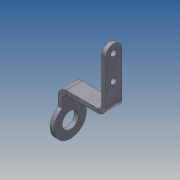
# Autodesk Inventor part: Gashebel_ra8846s
Saved by Autodesk Inventor 2021 (Build 250183000, 183)
## iProperties
Created: 2021-01-02
Part Number: Gashebel_ra8846s
Material: Aluminum 6061, geschweißt
Document SubType Name: Sheet Metal
Designer: Ricardo
Density: 2.7 g/cm^3
Sheet Metal Rule: Standard_mm
Appearance: Schweißnaht - Aluminum
Project: Motor
Description: Gashebel
Mass: 0.38312 g
Surface Area: 3.84459 cm^2
Volume: 0.141896 cm^3
Author: Sander
Revision Number: Rev00^
Autodesk Inventor part; units mm, degrees
ref_plane "YZ Plane" through (0, 0, 0) normal (1, 0, 0) x (0, 1, 0)
ref_plane "XZ Plane" through (0, 0, 0) normal (0, 1, 0) x (-1, 0, 0)
ref_plane "XY Plane" through (0, 0, 0) normal (0, 0, 1) x (1, 0, 0)
sketch "Skizze1" plane through (0, 0, 0) normal (0, 0, 1) x (1, 0, 0)
  line L0 (-38, 0) -> (11, 0)
  line L1 (0, -5.6) -> (0, 5.6)
  circle A0 centre (0, 0) radius 2
  line L2 (-3.4641, -2) -> (-29, -2)
  line L3 (-3.4641, 2) -> (-29, 2)
  arc A1 (-29, 2) -> (-29, -2) centre (-29, 0) ccw
  arc A2 (-3.4641, -2) -> (-3.4641, 2) centre (0, 0) ccw
  circle A3 centre (-29, 0) radius 0.75
  circle A4 centre (-23, 0) radius 0.75
  dimension "d0" = 4
  dimension "d1" = 4
  dimension "d2" = 6
  dimension "d3" = 1.5
  dimension "d4" = 1.5
  dimension "d5" = 2
  dimension "d6" = 29
  measures "d0" diameter of A0
  measures "d1" radius of A2
  measures "d2" distance of A1.centre A4.centre
  measures "d3" diameter of A4
  measures "d4" diameter of A3
  measures "d5" radius of A1
  measures "d6" distance from line of L1 A1.centre
extrude "Grobblech1" add sketch "Skizze1" along normal blind 1 contours A1 L3 A2 L1 A0 L0 A4 A3 | L0 A3 A4 A0 L1 A2 L2 A1 | A2 L0 A0 L1 | L1 A0 L0 A2
sketch "Skizze2" plane through (0, 0, 1) normal (0, 0, 1) x (1, 0, 0)
  circle A0 centre (-29, 0) radius 0.75 projected
  line L0 (-3.4641, -2) -> (-29, -2) projected
  line L1 (-29, 2) -> (-3.4641, 2) projected
  line L2 (-7, 2) -> (-7, -2)
  dimension "d8" = 22
  constraints: 2 end point, 2 point on line, 1 perpendicular
  measures "d8" distance from line of L2 A0.centre
fold "Falten1" angle 90 bend radius 1 thickness 1 k factor 0.44 line from (-7, 2, 1) to (-7, -2, 1) line at bend centre moving side (-1, 0, 0) folds toward (0, 0, 1)
sketch "Skizze3" plane through (-6.869, 0, 22.869) normal (1, 0, 0) x (0, 0, -1)
  line L0 (0, 2) -> (20.869, 2) projected
  arc A0 (0, 2) -> (0, -2) centre (0, 0) ccw projected
  line L1 (20.869, -2) -> (0, -2) projected
  line L2 (12, 2) -> (12, -2)
  point P0 (22.869, 0)
  dimension "d15" = 12
  constraints: 2 end point, 2 point on line, 1 perpendicular
  measures "d15" distance from line of L2 A0.centre
fold "Falten2" angle 90 bend radius 1 thickness 1 k factor 0.44 line from (-6.869, 2, 10.869) to (-6.869, -2, 10.869) line at bend centre moving side (0, 0, -1) folds toward (-1, 0, 0)
equation "\"d7\" = Thickness"
equation "\"d9\" = BendReliefWidth"
equation "\"d10\" = BendReliefDepth"
equation "\"d11\" = MinimumRemnant"
equation "\"d12\" = TransitionRadius"
equation "\"d14\" = BendRadius"
equation "\"d16\" = BendReliefWidth"
equation "\"d17\" = BendReliefDepth"
equation "\"d18\" = MinimumRemnant"
equation "\"d19\" = TransitionRadius"
equation "\"d21\" = BendRadius"
equation "\"BendRadius\" = Thickness"
equation "\"BendReliefWidth\" = Thickness"
equation "\"BendReliefDepth\" = 0.5 * Thickness"
equation "\"CornerReliefSize\" = 4 * Thickness"
equation "\"MinimumRemnant\" = 2 * Thickness"
equation "\"TransitionRadius\" = BendRadius"
equation "\"JacobiRadiusSize\" = BendRadius"
equation "\"GapSize\" = Thickness"
equation "\"Thickness\" = 1"
